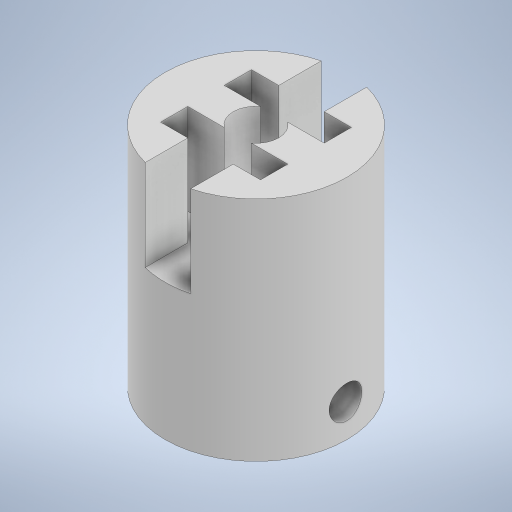
# Autodesk Inventor part: hub
Saved by Autodesk Inventor 2023 (Build 270158000, 158)
## iProperties
Created: 2025-12-21
Part Number: hub
Material: Generic
Document SubType Name: Modeling
Designer: Justin Pascual
Density: 1 g/cm^3
Appearance: Default
Author: Justin Pascual
Autodesk Inventor part; units mm, degrees
ref_plane "YZ Plane" through (0, 0, 0) normal (1, 0, 0) x (0, 1, 0)
ref_plane "XZ Plane" through (0, 0, 0) normal (0, 1, 0) x (-1, 0, 0)
ref_plane "XY Plane" through (0, 0, 0) normal (0, 0, 1) x (1, 0, 0)
sketch "Sketch1" plane through (0, 0, 0) normal (0, 1, 0) x (-1, 0, 0)
  circle A0 centre (0, 0) radius 12.7
  dimension "d0" = 25.4
  constraints: 1 centre point, 1 coincident
  measures "d0" diameter of A0
extrude "Extrusion1" add sketch "Sketch1" along normal blind 31.75
sketch "Sketch3" plane through (0, 31.75, 0) normal (0, 1, 0) x (1, 0, 0)
  circle A0 centre (0, 0) radius 12.7 projected
  line L0 (0, -12.7) -> (-3.175, -12.7)
  line L1 (-3.175, -12.7) -> (-3.175, -6.35)
  line L2 (-3.175, -6.35) -> (-6.985, -6.35)
  line L3 (-6.985, -6.35) -> (-6.985, -2.54)
  line L4 (-6.985, -2.54) -> (0, -2.54)
  line L5 (0, -12.7) -> (0, -2.54)
  line L6 (0, -12.7) -> (3.175, -12.7)
  line L7 (3.175, -12.7) -> (3.175, -6.35)
  line L8 (3.175, -6.35) -> (6.985, -6.35)
  line L9 (6.985, -6.35) -> (6.985, -2.54)
  line L10 (6.985, -2.54) -> (0, -2.54)
  point P0 (-3.175, -12.2967)
  point P1 (3.175, -12.2967)
  dimension "d3" = 3.175
  dimension "d4" = 6.35
  dimension "d5" = 3.81
  dimension "d6" = 3.81
  constraints: 22 end point, 4 symmetric about line, 3 horizontal, 2 perpendicular, 2 vertical, 2 other
  measures "d3" distance of L0.start L0.end
  measures "d4" distance of L0.end L1.end
  measures "d5" distance of L1.end L2.end
  measures "d6" distance of L2.end L3.end
extrude "Extrusion2" cut sketch "Sketch3" against normal blind 12.7 contours L1 L2 L3 L4 L5 A0 | A0 L5 L10 L9 L8 L7
mirror "Mirror1" about plane through (0, 0, 0) normal (0, 0, 1) of "Extrusion2"
sketch "Sketch4" plane through (0, 31.75, 0) normal (0, 1, 0) x (1, 0, 0)
  point P0 (0, 0)
  point P1 (0, 0)
  constraints: 1 coincident
hole "Hole1" at (0, 31.75, 0) direction (0, -1, 0) diameter 6.35 depth 12.7 clearance for "Flat Head Machine Screw" size "M6" standard "Ansi Metric M Profile"
sketch "Sketch5" plane through (0, 0, 0) normal (0, -1, 0) x (1, 0, 0)
  point P0 (0, 0)
  point P1 (0, 0)
  constraints: 1 coincident
hole "Hole2" at (0, 0, 0) direction (0, 1, 0) diameter 7.366 depth 12.7
sketch "Sketch8" plane through (0, 0, 0) normal (1, 0, 0) x (0, 1, 0)
  circle A0 centre (4.572, 0) radius 2.286
  line L0 (0, -12.7) -> (0, 12.7) projected
  point P0 (0, 0)
  dimension "d33" = 4.572
  dimension "d34" = 4.572
  constraints: 1 centre point
  measures "d33" diameter of A0
  measures "d34" distance from line of L0 A0.centre
extrude "Extrusion5" cut sketch "Sketch8" along normal mid plane 25.4
body "Solid1"
